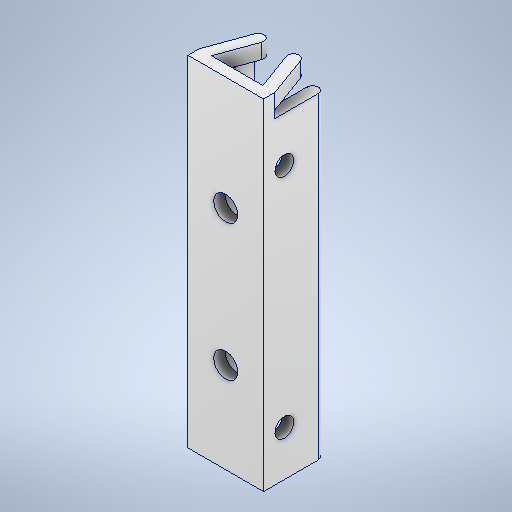
# Autodesk Inventor part: x_holder
Saved by Autodesk Inventor 2025 (Build 290162000, 162)
## iProperties
Created: 2024-04-25
Part Number: x_holder
Material: Hliník 6061
Document SubType Name: Modeling
Designer: rader
Density: 2.7 g/cm^3
Appearance: Hliník – plochý
Author: rader
Autodesk Inventor part; units mm, degrees
ref_plane "YZ Plane" through (0, 0, 0) normal (1, 0, 0) x (0, 1, 0)
ref_plane "XZ Plane" through (0, 0, 0) normal (0, 1, 0) x (-1, 0, 0)
ref_plane "XY Plane" through (0, 0, 0) normal (0, 0, 1) x (1, 0, 0)
sketch "Náčrt1" plane through (0, 0, 0) normal (0, 0, 1) x (1, 0, 0)
  line L0 (-7, 0) -> (7, 0) projected
  line L1 (0, 9.6) -> (0, -1.6) projected
  line L2 (-5, 8) -> (-5, 0)
  line L3 (-5, 0) -> (5, 0)
  line L4 (5, 0) -> (5, 8)
  line L5 (5, 8) -> (3.5, 8)
  line L6 (3.5, 8) -> (3.5, 1.5)
  line L7 (3.5, 1.5) -> (-3.5, 1.5)
  line L8 (-3.5, 1.5) -> (-3.5, 8)
  line L9 (-3.5, 8) -> (-5, 8)
  point P0 (0, 0)
  point P1 (-5, 0)
  dimension "d0" = 1.5
  dimension "d1" = 1.5
  dimension "d2" = 1.5
  dimension "d3" = 10
  dimension "d4" = 8
  dimension "d5" = 8
  constraints: 16 end point, 5 parallel, 2 perpendicular, 1 collinear, 1 vertical, 1 other
  measures "d0" distance of L4.end L5.end
  measures "d1" distance of L8.end L2.start
  measures "d2" distance between parallel lines of L3 L7
  measures "d3" distance of L2.end L3.end
  measures "d4" distance of L3.end L4.end
  measures "d5" distance of L2.start L2.end
extrude "Vysunutí1" add sketch "Náčrt1" along normal mid plane 42
sketch "Náčrt2" plane through (0, 0, 21) normal (0, 0, 1) x (1, 0, 0)
  line L0 (-5, 8) -> (-5, 0) projected
  line L1 (-5, 0) -> (5, 0) projected
  line L2 (5, 0) -> (5, 8) projected
  line L3 (5, 8) -> (3.5, 8) projected
  line L4 (3.5, 8) -> (3.5, 1.5) projected
  line L5 (3.5, 1.5) -> (-3.5, 1.5) projected
  line L6 (-3.5, 1.5) -> (-3.5, 8) projected
  line L7 (-3.5, 8) -> (-5, 8) projected
  line L8 (-5, 0) -> (5, 0)
  line L9 (5, 0) -> (5, 1.5)
  line L10 (5, 1.5) -> (-5, 1.5)
  line L11 (-5, 1.5) -> (-5, 0)
  point P0 (0, 0)
  constraints: 8 end point, 2 parallel, 1 collinear, 1 horizontal, 1 perpendicular, 1 point on line
extrude "Vysunutí2" add sketch "Náčrt2" along normal blind 1 contours L10 L5 L2 L1 L0
sketch "Náčrt3" plane through (0, 0, 22) normal (0, 0, 1) x (1, 0, 0)
  line L0 (-5, 1.5) -> (-5, 0) projected
  line L1 (-5, 0) -> (5, 0) projected
  line L2 (5, 0) -> (5, 1.5) projected
  line L3 (5, 1.5) -> (-5, 1.5) projected
  line L4 (5, 1.5) -> (5, 0)
  line L5 (5, 0) -> (-5, 0) projected
  line L6 (5, 0) -> (-5, 0)
  line L7 (-5, 0) -> (-5, 1.5)
  line L8 (-5, 1.5) -> (-2.7769, 7.608)
  line L9 (-5, 1.5) -> (1.5, 1.5) construction
  line L10 (-2.7769, 7.608) -> (-1.3673, 7.095)
  line L11 (-1.3673, 7.095) -> (-3.4037, 1.5)
  line L12 (0, 9.6) -> (0, -1.6) projected
  line L13 (5, 1.5) -> (2.7769, 7.608)
  line L14 (2.7769, 7.608) -> (1.3673, 7.095)
  line L15 (1.3673, 7.095) -> (3.4037, 1.5)
  line L16 (-3.4037, 1.5) -> (3.4037, 1.5)
  point P0 (0, 0)
  dimension "d10" = 6.5
  dimension "d11" = 70
  dimension "d12" = 1.5
  constraints: 22 end point, 4 collinear, 3 symmetric about line, 2 perpendicular, 1 equal length, 1 horizontal, 1 point on line
  measures "d10" distance of L0.start L8.end
  measures "d11" angle of L9 L8
  measures "d12" distance of L8.end L10.end
extrude "Vysunutí3" add sketch "Náčrt3" along normal blind 2
fillet "Zaoblení1" radius 0.75 8 edges at (-5, 8, 0) (-3.5, 8, 0) (3.5, 8, 0) (5, 8, 0) (1.3673, 7.095, 23) (2.7769, 7.608, 23) (-2.7769, 7.608, 23) (-1.3673, 7.095, 23)
sketch "Náčrt4" plane through (5, 0, 24) normal (1, 0, 0) x (0, 0, -1)
  line L0 (3, 7.25) -> (45, 7.25) projected
  line L1 (3, 1.5) -> (3, 7.25) projected
  line L2 (3, 1.5) -> (2, 1.5) projected
  line L3 (2, 1.5) -> (0, 1.5) projected
  line L4 (0, 0) -> (0, 1.5) projected
  line L5 (45, 0) -> (0, 0) projected
  line L6 (45, 7.25) -> (45, 0) projected
  point P0 (24, 0)
  point P1 (9, 2.75)
  point P2 (39, 2.75)
  dimension "d16" = 2.75
  dimension "d17" = 2.75
  dimension "d18" = 6
  dimension "d19" = 30
  measures "d16" distance from line of L5 point (9, 2.75)
  measures "d17" distance from line of L5 point (39, 2.75)
  measures "d18" distance from line of L6 point (39, 2.75)
  measures "d19" distance of point (9, 2.75) point (39, 2.75)
hole "Díra1" at (5, 2.75, 15) at (5, 2.75, -15) direction (-1, 0, 0) diameter 2.5 end through all
sketch "Náčrt5" plane through (-3.5, 1.5, -21) normal (0, 1, 0) x (1, 0, 0)
  line L0 (7, 0) -> (7, -6) projected
  line L1 (0, 0) -> (7, 0) projected
  line L2 (0, 0) -> (0, -6) projected
  line L3 (0, -6) -> (0, -36) projected
  line L4 (0, -36) -> (0, -42) projected
  line L5 (-1.5, -42) -> (0, -42) projected
  line L6 (-1.5, -42) -> (-1.5, -43) projected
  line L7 (0.0963, -43) -> (-1.5, -43) projected
  line L8 (0.0963, -43) -> (0.0963, -45) projected
  line L9 (6.9037, -45) -> (0.0963, -45) projected
  line L10 (6.9037, -43) -> (6.9037, -45) projected
  line L11 (8.5, -43) -> (6.9037, -43) projected
  line L12 (8.5, -42) -> (8.5, -43) projected
  line L13 (7, -42) -> (8.5, -42) projected
  line L14 (7, -36) -> (7, -42) projected
  line L15 (7, -6) -> (7, -36) projected
  line L16 (10.5, -21) -> (-3.5, -21) projected
  line L17 (3.5, 9) -> (3.5, -54) projected
  point P0 (3.5, -21)
  point P1 (3.5, -12)
  point P2 (3.5, -30)
  dimension "d27" = 12
  dimension "d28" = 18
  constraints: 2 point on line
  measures "d27" distance from line of L1 point (3.5, -12)
  measures "d28" distance of point (3.5, -30) point (3.5, -12)
hole "Díra2" at (0, 1.5, -9) at (0, 1.5, 9) direction (0, -1, 0) diameter 3.2 end through all
